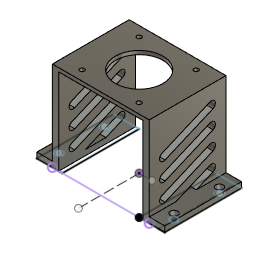
stepper_stand v8 (Autodesk Fusion 360 design; units mm, degrees)
Autodesk Fusion 360 part; units mm, degrees
sketch "Sketch1" plane through (0, 0, 0) normal (0, 0, 1) x (1, 0, 0)
  circle A0 centre (0, 0) radius 13
  line L0 (0, 0) -> (0, -24.6468) construction
  line L1 (0, 0) -> (22.786, 0) construction
  line L2 (-21, 0) -> (-21, -21)
  line L3 (-21, -21) -> (0, -21)
  line L4 (-15.6, -21) -> (-15.6, -15.6) construction
  line L5 (-15.6, -15.6) -> (-21, -15.6) construction
  circle A1 centre (-15.6, -15.6) radius 1.25
  line L6 (21, -21) -> (0, -21)
  line L7 (21, 0) -> (21, -21)
  circle A2 centre (15.6, -15.6) radius 1.25
  line L8 (21, 0) -> (21, 21)
  line L9 (21, 21) -> (0, 21)
  circle A3 centre (15.6, 15.6) radius 1.25
  line L10 (-21, 21) -> (0, 21)
  circle A4 centre (-15.6, 15.6) radius 1.25
  line L11 (-21, 0) -> (-21, 21)
  line L12 (-21, 21) -> (-22.5, 21)
  line L13 (-21, -21) -> (-22.5, -21)
  line L14 (-22.5, 21) -> (-22.5, -21)
  line L15 (22.5, 21) -> (22.5, -21)
  line L16 (21, 21) -> (22.5, 21)
  line L17 (21, -21) -> (22.5, -21)
  dimension "d14" = 26
  dimension "d15" = 21
  dimension "d16" = 21
  dimension "d17" = 5.4
  dimension "d18" = 5.4
  dimension "d19" = 2.5
  dimension "d34" = 1.5
  dimension "d35" = 1.5
  constraint coincident A0.centre L0.start
  constraint vertical L0
  constraint perpendicular L0 L1
  constraint vertical L2
  constraint horizontal L3
  constraint vertical L4
  constraint horizontal L5
  constraint coincident L4.end L5.start
  constraint symmetric L0 L2.start L7.start
  constraint symmetric L0 L2.end L6.start
  constraint symmetric L0 L3.end L6.end
  constraint symmetric L0 A1 A2
  constraint symmetric L1 L2.start L11.start
  constraint symmetric L1 L2.end L10.start
  constraint symmetric L1 L3.end L9.end
  constraint symmetric L1 A1 A4
  constraint symmetric L1 L6.start L8.end
  constraint symmetric L1 L7.start L8.start
  constraint symmetric L1 A2 A3
  constraint perpendicular L11 L12
  constraint perpendicular L2 L13
  constraint symmetric L0 L10.start L8.end
  constraint symmetric L0 L12.end L15.start
  constraint symmetric L0 L13.end L15.end
  measures "d14" diameter of A0
  measures "d15" distance of A0.centre L2.start
  measures "d16" distance of A0.centre L3.end
  measures "d17" distance of L2.end L4.start
  measures "d18" distance of L2.end L5.end
  measures "d19" diameter of A1
  measures "d34" distance of L10.start L12.end
  measures "d35" distance of L2.end L13.end
extrude "Extrude5" add sketch "Sketch1" along normal blind 2 contours L2 L3 L6 L7 L8 L9 L10 L11
sketch "Sketch5" plane through (21, 0, 0) normal (1, 0, 0) x (0, 1, 0)
  line L0 (-21, 0) -> (21, 0)
  line L1 (21, 0) -> (21, 2)
  line L2 (21, 2) -> (-21, 2)
  line L3 (-21, 2) -> (-21, 0)
  line L4 (-21, 2) -> (21, 2)
  line L5 (21, 2) -> (21, -47)
  line L6 (21, -47) -> (-21, -47)
  line L7 (-21, -47) -> (-21, 2)
  dimension "d22" = 49
  constraint horizontal L4
  constraint vertical L5
  constraint horizontal L6
  constraint vertical L7
  constraint coincident L2.end L3.start
  measures "d22" distance of L2.end L6.end
extrude "Extrude6" add sketch "Sketch5" along normal blind 5.5
sketch "Sketch6" plane through (-21, 0, 0) normal (-1, 0, 0) x (0, -1, 0)
  line L0 (-21, 0) -> (21, 0)
  line L1 (21, 0) -> (21, 2)
  line L2 (21, 2) -> (-21, 2)
  line L3 (-21, 2) -> (-21, 0)
  line L4 (-21, 2) -> (21, 2)
  line L5 (21, 2) -> (21, -47)
  line L6 (21, -47) -> (-21, -47)
  line L7 (-21, -47) -> (-21, 2)
  point P0 (21, -47)
  constraint horizontal L4
  constraint vertical L5
  constraint horizontal L6
  constraint vertical L7
  constraint coincident P0 L5.end
  constraint coincident L2.end L3.start
extrude "Extrude7" add sketch "Sketch6" along normal blind 5.5
sketch "Sketch7" plane through (0, 0, -47) normal (0, 0, -1) x (1, 0, 0)
  line L0 (-21, -21) -> (-21, 21)
  line L1 (-21, 21) -> (-26.5, 21)
  line L2 (-26.5, 21) -> (-26.5, -21)
  line L3 (-26.5, -21) -> (-21, -21)
  line L4 (21, 21) -> (35, 21)
  line L5 (35, 21) -> (35, -21)
  line L6 (35, -21) -> (21, -21)
  line L7 (21, -21) -> (21, 21)
  line L8 (26.5, 21) -> (-26.5, 21)
  line L9 (0, 0) -> (0, 33.2461) construction
  line L10 (35, 21) -> (31.5, 21)
  line L11 (31.5, 21) -> (31.5, -21) construction
  circle A0 centre (31.5, 12.4587) radius 2
  line L12 (0, 0) -> (6.9682, 0) construction
  circle A1 centre (31.5, -12.4587) radius 2
  line L13 (-21, 21) -> (-35, 21)
  line L14 (-21, -21) -> (-21, 21)
  line L15 (-35, 21) -> (-35, -21)
  circle A2 centre (-31.5, 12.4587) radius 2
  circle A3 centre (-31.5, -12.4587) radius 2
  line L16 (-35, -21) -> (-21, -21)
  point P0 (21, 21)
  dimension "d27" = 14
  dimension "d28" = 3.5
  dimension "d29" = 4
  constraint horizontal L4
  constraint vertical L5
  constraint horizontal L6
  constraint vertical L7
  constraint coincident P0 L4.start
  constraint coincident L9.start L12.start
  constraint perpendicular L8 L9
  constraint perpendicular L5 L10
  constraint coincident L6 L11.end
  constraint perpendicular L6 L11
  constraint coincident L11 A0.centre
  constraint horizontal L12
  constraint symmetric A0 L12 A1
  constraint symmetric P0 L9 L0.end
  constraint symmetric L4.end L9 L13.end
  constraint symmetric L5.end L9 L15.end
  constraint symmetric L6.end L9 L0.start
  constraint symmetric L9 A0 A2
  constraint symmetric L9 A1 A3
  measures "d27" distance of P0 L4.end
  measures "d28" distance of L4.end L10.end
  measures "d29" diameter of A0
extrude "Extrude8" add sketch "Sketch7" against normal blind 3
sketch "Sketch8" plane through (-26.5, 0, 0) normal (-1, 0, 0) x (0, -1, 0)
  line L0 (21, -44) -> (21, 2)
  line L1 (21, 2) -> (-21, 2)
  line L2 (-21, 2) -> (-21, -44)
  line L3 (-13.922, -10.1005) -> (12.3505, -21.3101)
  arc A0 (12.3505, -21.3101) -> (14.056, -17.313) centre (13.2033, -19.3115) ccw
  line L4 (14.056, -17.313) -> (-12.2165, -6.1034)
  arc A1 (-12.2165, -6.1034) -> (-13.922, -10.1005) centre (-13.0693, -8.1019) ccw
  line L5 (-15.0678, -7.2492) -> (15.2018, -20.1642) construction
  line L6 (-13.922, -20.1005) -> (12.3505, -31.3101)
  arc A2 (-12.2165, -16.1034) -> (-13.922, -20.1005) centre (-13.0693, -18.1019) ccw
  line L7 (14.056, -27.313) -> (-12.2165, -16.1034)
  arc A3 (12.3505, -31.3101) -> (14.056, -27.313) centre (13.2033, -29.3115) ccw
  line L8 (14.056, -37.313) -> (-12.2165, -26.1034)
  line L9 (-13.922, -30.1005) -> (12.3505, -41.3101)
  arc A4 (12.3505, -41.3101) -> (14.056, -37.313) centre (13.2033, -39.3115) ccw
  arc A5 (-12.2165, -26.1034) -> (-13.922, -30.1005) centre (-13.0693, -28.1019) ccw
  line L10 (-13.922, -40.1005) -> (12.3505, -51.3101)
  line L11 (14.056, -47.313) -> (-12.2165, -36.1034)
  arc A6 (-12.2165, -36.1034) -> (-13.922, -40.1005) centre (-13.0693, -38.1019) ccw
  arc A7 (12.3505, -51.3101) -> (14.056, -47.313) centre (13.2033, -49.3115) ccw
  line L12 (-21, -44) -> (21, -44)
  point P0 (15.2018, -30.1642)
  constraint tangent L3 A0
  constraint tangent A0 L4
  constraint parallel L3 L4
  constraint tangent L4 A1
  constraint tangent L3 A1
  constraint midpoint A1 L5.start
  constraint midpoint A0 L5.end
  constraint tangent L6 A3
  constraint tangent L7 A3
  constraint parallel L6 L7
  constraint tangent A2 L7
  constraint tangent L6 A2
  constraint midpoint P0 A3
  constraint tangent L9 A4
  constraint tangent L8 A4
  constraint parallel L8 L9
  constraint tangent L8 A5
  constraint tangent L9 A5
  constraint tangent L10 A7
  constraint tangent L11 A7
  constraint parallel L10 L11
  constraint tangent L11 A6
  constraint tangent L10 A6
extrude "Extrude9" cut sketch "Sketch8" against normal up to surface (53 mm away) contours L10 L11 A6 L12 | L10 L11 A7 L12 | L3 A0 L4 A1 | L6 A2 L7 A3 | L8 L9 A4 A5
move_face "OffsetFaces1" offset -1.5 1 faces at (-21, -7.6131, -7.8054)
move_face "OffsetFaces2" offset -1.5 1 faces at (21, -7.6131, -7.8054)
move_face "OffsetFaces3" offset -0.5 1 faces at (-22.5, -7.6131, -7.8054)
move_face "OffsetFaces4" offset -0.5 1 faces at (22.5, -7.6131, -7.8054)
move_face "OffsetFaces5" offset 3.5 1 faces at (26.5, -7.2875, -46)
move_face "OffsetFaces6" offset 3.5 1 faces at (-26.5, -7.2875, -46)
